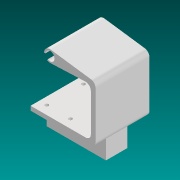
# Autodesk Inventor part: 链接板2
Saved by Autodesk Inventor 2021 (Build 250183000, 183)
## iProperties
Created: 2025-04-17
Part Number: 链接板2
Material: 常规
Document SubType Name: Modeling
Designer: 86155
Density: 1 g/cm^3
Appearance: 默认
Author: 86155
Autodesk Inventor part; units mm, degrees
ref_plane "YZ Plane" through (0, 0, 0) normal (1, 0, 0) x (0, 1, 0)
ref_plane "XZ Plane" through (0, 0, 0) normal (0, 1, 0) x (-1, 0, 0)
ref_plane "XY Plane" through (0, 0, 0) normal (0, 0, 1) x (1, 0, 0)
sketch "草图1" plane through (0, 0, 0) normal (0, 0, 1) x (1, 0, 0)
  circle A0 centre (0, 41) radius 4.25 projected
  circle A1 centre (0, 41) radius 4.25
  line L0 (0, 41) -> (-2.75, 36.2369)
  line L1 (0, 41) -> (5.5, 41) construction
  line L2 (0, 41) -> (-5.5, 41)
  line L3 (0.7501, 46.4486) -> (42.3728, 40.7189)
  line L4 (-15, 3) -> (-15, 6) projected
  line L5 (-15, 6) -> (-18, 6) projected
  line L6 (-18, 6) -> (-18, -8) projected
  line L7 (-4, -8) -> (-18, -8) projected
  line L8 (-4, -6) -> (-4, -8) projected
  line L9 (-4, -6) -> (4, -6) projected
  line L10 (4, -6) -> (4, -8) projected
  line L11 (18, -8) -> (4, -8) projected
  line L12 (18, 6) -> (18, -8) projected
  line L13 (18, 6) -> (15, 6) projected
  line L14 (15, 6) -> (15, 3) projected
  line L15 (15, 3) -> (13.5, 3) projected
  line L16 (13.5, 3) -> (13.5, 2) projected
  line L17 (13.5, 2) -> (15, 2) projected
  line L18 (15, 2) -> (15, -2) projected
  line L19 (15, -2) -> (-15, -2) projected
  line L20 (-15, -2) -> (-15, 2) projected
  line L21 (-15, 2) -> (-13.5, 2) projected
  line L22 (-13.5, 2) -> (-13.5, 3) projected
  line L23 (-13.5, 3) -> (-15, 3) projected
  line L24 (-18, -8) -> (18, -8)
  line L25 (18, -8) -> (18, -12)
  line L26 (18, -12) -> (-18, -12)
  line L27 (-18, -12) -> (-18, -8)
  line L28 (18, -12) -> (42.3728, -12)
  line L29 (42.3728, -12) -> (42.3728, 40.7189)
  line L30 (18, -8) -> (38, -8)
  line L31 (38, -8) -> (38, 37.0777)
  line L32 (0.2288, 35.5048) -> (38, 37.0777)
  arc A2 (-2.75, 36.2369) -> (0.2288, 35.5048) centre (0, 41) ccw
  arc A3 (0.7501, 46.4486) -> (-5.5, 41) centre (0, 41) ccw
  point P0 (0, 0)
  point P1 (-4.25, 41)
  point P2 (-2.125, 37.3194)
  dimension "d1" = 120
  dimension "d2" = 4
  dimension "d3" = 20
  constraints: 26 end point, 4 horizontal, 4 point on circle, 3 centre point, 3 perpendicular, 2 coincident, 2 parallel, 2 tangent, 1 concentric, 1 equal length, 1 point on line
  measures "d1" angle of L0 L1
  measures "d2" distance of L24.end L25.end
  measures "d3" distance of L24.end L30.end
extrude "拉伸1" add sketch "草图1" against normal blind 50 contours A0 L2 A3 L3 L29 L28 L25 L30 L31 L32 A2 L0 | L26 L27 L7 L24 L11 L25
fillet "圆角1" radius 5 2 edges at (38, 37.0777, -25) (42.3728, 40.7189, -25)
fillet "圆角2" radius 5 2 edges at (38, -8, -25) (42.3728, -12, -25)
sketch "草图2" plane through (-18, -12, -50) normal (0, -1, 0) x (1, 0, 0)
  line L0 (0, 50) -> (55.3728, 50) projected
  line L1 (0, 50) -> (0, 0) projected
  line L2 (55.3728, 0) -> (0, 0) projected
  point P0 (18, 50)
  point P1 (7, 42)
  point P2 (7, 8)
  point P3 (29, 42)
  point P4 (29, 8)
  dimension "d8" = 8
  dimension "d9" = 7
  dimension "d10" = 8
  dimension "d11" = 22
  measures "d8" distance from line of L0 point (7, 42)
  measures "d9" distance from line of L1 point (7, 42)
  measures "d10" distance from line of L2 point (7, 8)
  measures "d11" distance of point (29, 42) point (7, 42)
hole "孔1" at (-11, -12, -8) at (-11, -12, -42) at (11, -12, -8) at (11, -12, -42) direction (0, 1, 0) diameter 3.242 depth 4 countersink diameter 4 countersink angle 90 thread size "M4x0.7" designation "M4" class "6H" standard "GB Metric profile"
sketch "草图3" plane through (-18, -12, -50) normal (0, -1, 0) x (1, 0, 0)
  line L0 (0, 50) -> (0, 0) projected
  line L1 (0, 35) -> (55, 35)
  line L2 (55, 35) -> (55, 15)
  line L3 (55, 15) -> (0, 15)
  line L4 (0, 15) -> (0, 35)
  line L5 (0, 50) -> (55.3728, 50) projected
  point P0 (18, 50)
  point P1 (0, 15)
  dimension "d19" = 55
  dimension "d20" = 20
  dimension "d21" = 15
  constraints: 8 end point, 2 parallel, 1 horizontal, 1 perpendicular, 1 point on line
  measures "d19" distance of L2.end L3.end
  measures "d20" distance of L1.end L2.end
  measures "d21" distance between parallel lines of L5 L1
extrude "拉伸2" add sketch "草图3" along normal blind 20
